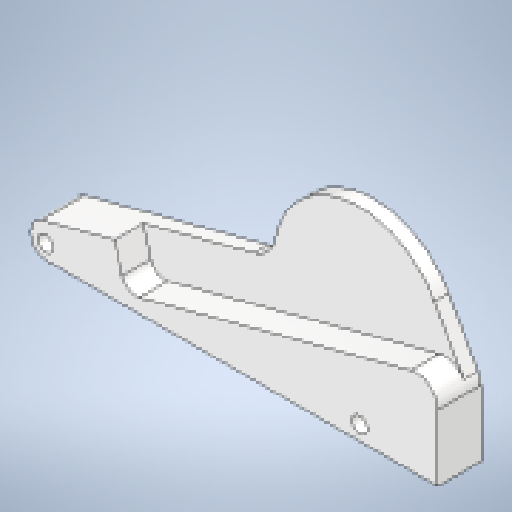
# Autodesk Inventor part: Uprights
Saved by Autodesk Inventor 2023.2 (Build 272271000, 271)
## iProperties
Created: 2024-01-11
Part Number: Uprights
Material: UHMW, White
Document SubType Name: Modeling
Designer: Nathan Cai
Mass: 11.9669 g
Surface Area: 63.9839 cm^2
Volume: 12.7307 cm^3
Density: 0.94 g/cm^3
Appearance: Smooth - White
Angle_Mount: 105.00 deg
Rail_Offset: 1.438 in
Author: Nathan Cai
Autodesk Inventor part; units mm, degrees
ref_plane "YZ Plane" through (0, 0, 0) normal (1, 0, 0) x (0, 1, 0)
ref_plane "XZ Plane" through (0, 0, 0) normal (0, 1, 0) x (-1, 0, 0)
ref_plane "XY Plane" through (0, 0, 0) normal (0, 0, 1) x (1, 0, 0)
sketch "Sketch2" plane through (0, 0, 0) normal (0, 0, 1) x (1, 0, 0)
  circle A0 centre (0, 0) radius 3.175 construction
  circle A1 centre (0, 0) radius 7.9375 construction
  line L0 (-24.9815, -53.975) -> (30.0677, -53.975)
  line L1 (-24.9815, -53.975) -> (-36.2864, -11.7845) construction
  line L2 (-36.2864, -11.7845) -> (-3.9688, 6.8741) construction
  line L3 (20.5427, -47.625) -> (-13.5349, -47.625)
  line L4 (-13.5349, -47.625) -> (-22.3476, -14.7355) construction
  line L5 (-22.3476, -14.7355) -> (-5.9414, -5.2634) construction
  line L6 (-18.5621, -41.1307) -> (-23.4926, -22.7298) construction
  line L7 (-23.4926, -22.7298) -> (-29.6262, -24.3733) construction
  line L8 (-29.6262, -24.3733) -> (-24.6957, -42.7742) construction
  line L9 (-24.6957, -42.7742) -> (-18.5621, -41.1307) construction
  line L10 (-18.5621, -41.1307) -> (-29.6262, -24.3733) construction
  line L11 (-23.4926, -22.7298) -> (-24.6957, -42.7742) construction
  circle A2 centre (-29.6262, -24.3733) radius 1.7526 construction
  circle A3 centre (-24.6957, -42.7742) radius 1.7526 construction
  circle A4 centre (-21.0273, -31.9303) radius 1.7526 construction
  line L12 (25.3052, -45.5804) -> (25.3052, -53.975)
  circle A5 centre (25.3052, -39.2375) radius 1.7526
  line L13 (0, 0) -> (-58.6646, -15.7191) construction
  line L14 (-24.0941, -32.752) -> (-30.6681, -8.2175) construction
  circle A6 centre (25.3052, -39.2375) radius 4.7625
  line L15 (30.0677, -39.2375) -> (30.0677, -53.975)
  line L16 (20.5427, -39.2375) -> (20.5427, -47.625)
  line L17 (-30.2278, -34.3955) -> (-17.9605, -31.1085) construction
  line L18 (-24.9815, -53.975) -> (-113.8815, -53.975)
  circle A7 centre (-9.9632, -48.6877) radius 1.7526
  line L19 (-9.9632, -48.6877) -> (-25.2973, -52.7964) construction
  line L20 (25.3052, -39.2375) -> (24.0725, -34.6373)
  line L21 (-31.2313, -30.6503) -> (-77.8688, -47.625) construction
  line L22 (-77.8688, -47.625) -> (-26.6829, -47.625) construction
  line L23 (-9.9632, -48.6877) -> (-10.4168, -46.9948) construction
  circle A8 centre (25.3052, -39.2375) radius 1.7526
  circle A9 centre (25.3052, -39.2375) radius 4.7625
  line L24 (17.994, -39.5531) -> (8.9547, -5.8181) construction
  line L25 (8.9547, -5.8181) -> (-22.4801, -14.241) construction
  line L26 (-22.4801, -14.241) -> (-13.4409, -47.976) construction
  line L27 (-0.2817, -44.45) -> (17.994, -39.5531) construction
  line L28 (17.994, -39.5531) -> (-22.4801, -14.241) construction
  line L29 (8.9547, -5.8181) -> (-13.4409, -47.976) construction
  line L30 (6.9477, 3.8384) -> (29.4738, -36.9345)
  line L31 (2.0544, -7.667) -> (8.9547, -5.8181) construction
  circle A10 centre (-9.9632, -48.6877) radius 4.7625
  line L32 (-0.2817, -44.45) -> (-14.3857, -44.45) construction
  line L33 (-113.8815, -53.975) -> (-32.8811, -24.4933) construction
  circle A11 centre (-54.7623, -40.9695) radius 1.7526 construction
  circle A12 centre (-54.7623, -40.9695) radius 7.9375 construction
  line L34 (-54.7623, -40.9695) -> (-56.8404, -33.2138) construction
  line L35 (-25.8322, -50.8) -> (-105.1582, -50.8) construction
  circle A13 centre (-57.15, -50.8) radius 1.7526
  circle A14 centre (-66.675, -50.8) radius 1.7526 construction
  circle A15 centre (-76.2, -50.8) radius 1.7526 construction
  circle A16 centre (-85.725, -50.8) radius 1.7526 construction
  circle A17 centre (12.7, -50.8) radius 1.7526
  line L36 (-2.2431, -26.897) -> (20.5536, -20.7887) construction
  line L37 (25.3052, -39.2375) -> (-9.9632, -48.6877) construction
  line L38 (26.5378, -43.8377) -> (-8.7306, -53.2879)
  line L39 (-48.0967, -53.975) -> (24.0725, -34.6373)
  arc A18 (26.5378, -43.8377) -> (24.0725, -34.6373) centre (25.3052, -39.2375) ccw
  arc A19 (-11.1958, -44.0874) -> (-8.7306, -53.2879) centre (-9.9632, -48.6877) ccw
  line L40 (-36.2475, -50.8) -> (-36.2475, -53.975) construction
  line L41 (-36.2475, -50.8) -> (-38.7127, -41.5996) construction
  line L42 (-38.7127, -41.5996) -> (-84.8985, -53.975)
  circle A20 centre (-37.0692, -47.7332) radius 3.175
  line L43 (-41.7795, -42.4213) -> (-39.3143, -51.6218)
  line L44 (-38.7127, -41.5996) -> (22.9264, -25.0834)
  arc A21 (22.9264, -25.0834) -> (-12.7947, -34.6548) centre (6.2519, -34.2957) ccw
  line L45 (-39.3143, -51.6218) -> (27.6718, -33.6729) construction
  circle A22 centre (-57.15, -50.8) radius 3.175
  line L46 (-60.325, -50.8) -> (-60.325, -47.3906)
  point P0 (30.0677, -39.2375)
  point P1 (-24.0941, -32.752)
  point P2 (-2.2431, -26.897)
  point P3 (-12.1309, -47.625)
  point P4 (-15.5208, -47.3441)
  point P5 (-14.3857, -44.45)
  point P6 (-9.6568, -46.9621)
  point P7 (-9.6568, -46.9621)
  point P8 (-48.0301, -36.7646)
  point P9 (-59.0876, -47.625)
  point P10 (-62.6223, -42.0757)
  point P11 (-50.4369, -47.625)
  point P12 (0.6918, 7.9073)
  point P13 (7.671, -43.9626)
  point P14 (26.5378, -43.8377)
  point P15 (-40.136, -48.5549)
  point P16 (-57.15, -53.975)
  dimension "d40" = 3.5052
  dimension "d6" = 6.35
  dimension "d7" = 15.875
  dimension "Angle_Mount" = 105
  dimension "d17" = 105
  dimension "d19" = 9.525
  dimension "d20" = 12.7
  dimension "d24" = 19.05
  dimension "d25" = 6.35
  dimension "d26" = 3.5052
  dimension "d27" = 3.5052
  dimension "d28" = 3.5052
  dimension "d29" = 6.35
  dimension "d33" = 3.5052
  dimension "d35" = 31.75
  dimension "d37" = 9.525
  dimension "d38" = 25.4
  dimension "d39" = 53.975
  dimension "d41" = 44.45
  dimension "Rail_Offset" = 36.5125
  dimension "d45" = 6.35
  dimension "d48" = 22.225
  dimension "d49" = 3.5052
  dimension "d51" = 9.525
  dimension "d52" = 32.5438
  dimension "d53" = 34.925
  dimension "d54" = 9.525
  dimension "d56" = 9.525
  dimension "d58" = 6.35
  dimension "d60" = 20
  dimension "d61" = 88.9
  dimension "d69" = 31.75
  dimension "d71" = 3.5052
  dimension "d72" = 15.875
  dimension "d74" = 3.175
  dimension "d75" = 3.5052
  dimension "d76" = 57.15
  dimension "d79" = 9.525
  dimension "d84" = 3.5052
  dimension "d85" = 69.85
  dimension "d106" = 3.175
  dimension "d107" = 9.525
  dimension "d109" = 6.35
  dimension "d113" = 19.05
  dimension "d122" = 9.525
  constraints: 96 end point, 36 point on line, 21 centre point, 17 point on circle, 15 parallel, 14 perpendicular, 13 tangent, 11 coincident, 9 midpoint, 4 horizontal, 2 concentric, 2 vertical, 1 collinear, 12 other
  measures "d6" diameter of A0
  measures "d7" diameter of A1
  measures "Angle_Mount" angle of L0 L1
  measures "d17" angle of L2 L1
  measures "d19" distance between parallel lines of L2 L5
  measures "d20" distance between parallel lines of L1 L4
  measures "d24" distance of L6.start L6.end
  measures "d25" distance of L7.end L6.end
  measures "d26" diameter of A2
  measures "d27" diameter of A3
  measures "d28" diameter of A4
  measures "d29" distance between parallel lines of L0 L3
  measures "d33" diameter of A5
  measures "d35" distance from line of point (0, 0) L14
  measures "d37" diameter of A6
  measures "d38" distance between parallel lines of L13 L17
  measures "d39" distance from line of L0 point (0, 0)
  measures "d41" distance between parallel lines of L13 L19
  measures "Rail_Offset" distance from line of L19.start L20
  measures "d45" distance between parallel lines of L18 L22
  measures "d48" distance from line of point (0, 0) L23
  measures "d49" diameter of A8
  measures "d51" diameter of A9
  measures "d52" distance between parallel lines of L24 L26
  measures "d53" distance between parallel lines of L27 L25
  measures "d54" diameter of A10
  measures "d56" distance between parallel lines of L0 L32
  measures "d58" distance between parallel lines of L21 L33
  measures "d60" angle of L22 L21
  measures "d61" distance of L0.start L18.end
  measures "d69" distance between parallel lines of L14 L34
  measures "d71" diameter of A11
  measures "d72" diameter of A12
  measures "d74" distance between parallel lines of L22 L35
  measures "d75" diameter of A13
  measures "d76" horizontal distance of A13.centre L13.start
  measures "d79" distance of A13.centre A14.centre
  measures "d84" diameter of A17
  measures "d85" distance of A13.centre A17.centre
  measures "d106" distance from line of L18 L40.start
  measures "d107" distance of L40.start L41.end
  measures "d109" diameter of A20
  measures "d113" radius of A21
  measures "d122" distance between parallel lines of L45 L44
extrude "Extrusion2" add sketch "Sketch2" along normal blind 9.525 contours L18 L39 A10 L38 L3 L16 A6 L15 L0 | L18 A22 L46 L42 L43 L39 | A22 | A6 | L38 L16 A6 | A10 | L39 A6 L16 L38 L3 A10 | L16 L3 L38 | A10 L3 L38 | A7 L3 | L3 A7 | A5
extrude "Extrusion3" add sketch "Sketch2" along normal blind 3.175 contours L43 A20 L39 | A20 L43 L42 L44 L30 A6 L39 | A20 | L38 L16 A6 | A10 | L39 A6 L16 L38 L3 A10 | L44 A21 | A10 L3 L38 | A7 L3 | L3 A7
fillet "Fillet6" radius 6.35 3 edges at (22.9264, -25.0834, 1.5875) (-12.7947, -34.6548, 1.5875) (29.4738, -36.9345, 1.5875)
fillet "Fillet7" radius 3.175 2 edges at (-39.3143, -51.6218, 6.35) (-60.325, -47.3906, 4.7625)
body "Solid2"
